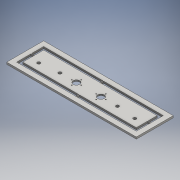
# Autodesk Inventor part: side-UPDATED
Saved by Autodesk Inventor 2,016 (Build 200138000, 138)
## iProperties
Created: 2016-10-15
Part Number: side-UPDATED
Material: Generic
Document SubType Name: Modeling
Designer: Kevin G
Density: 1 g/cm^3
Appearance: Default
Author: Kevin G
Autodesk Inventor part; units mm, degrees
note: some values were not read from the file. Chosen so that the rebuilt part matches the saved one: direction of "Emboss2".
ref_plane "YZ Plane" through (0, 0, 0) normal (1, 0, 0) x (0, 1, 0)
ref_plane "XZ Plane" through (0, 0, 0) normal (0, 1, 0) x (-1, 0, 0)
ref_plane "XY Plane" through (0, 0, 0) normal (0, 0, 1) x (1, 0, 0)
sketch "Sketch1" plane through (0, 0, 0) normal (0, 0, 1) x (1, 0, 0)
  line L0 (-270.2344, -114.33) -> (-270.2344, -13.08)
  circle A0 centre (-227.9995, -79.405) radius 7.5
  circle A1 centre (-134.4524, -69.88) radius 7.5
  circle A2 centre (-54.3408, -69.88) radius 15.875
  circle A3 centre (-54.3408, -46.8612) radius 2.3813
  circle A4 centre (-31.322, -69.88) radius 2.3813
  circle A5 centre (-77.3595, -69.88) radius 2.3813
  circle A6 centre (-54.3408, -92.8987) radius 2.3813
  line L1 (-270.2344, -13.08) -> (5.175, -13.08)
  line L2 (-270.2344, -114.33) -> (5.1968, -114.33)
  line L3 (280.6281, -114.33) -> (280.6281, -13.08)
  line L4 (280.6281, -13.08) -> (5.175, -13.08)
  line L5 (280.6281, -114.33) -> (5.1968, -114.33)
  line L6 (-285.2344, 1.92) -> (295.5844, 1.92)
  line L7 (295.5844, 1.92) -> (295.5844, -129.33)
  line L8 (295.5844, -129.33) -> (-285.2344, -129.33)
  line L9 (-285.2344, -129.33) -> (-285.2344, 1.92)
  line L10 (-59, 1.92) -> (-59, 25.92)
  line L11 (-285.2344, -38) -> (-309.2344, -38)
  line L12 (-43, -129.33) -> (-43, -153.33)
  line L13 (295.5844, -72.2612) -> (319.5844, -72.2612)
  line L14 (-309.2344, 25.92) -> (319.6281, 25.92)
  line L15 (319.6281, 25.92) -> (319.6281, -153.33)
  line L16 (319.6281, -153.33) -> (-309.2344, -153.33)
  line L17 (-309.2344, -153.33) -> (-309.2344, 25.92)
  line L18 (2, -13.08) -> (2, 1.92)
  line L19 (5.175, -13.08) -> (5.175, 1.92)
  line L20 (2, -129.33) -> (2, -114.33)
  line L21 (-285.2344, -56.825) -> (-270.2344, -56.825)
  line L22 (-285.2344, -60) -> (-270.2344, -60)
  line L23 (280.6281, -56.825) -> (295.5844, -56.825)
  line L24 (5.1968, -114.33) -> (5.175, -129.33)
  line L25 (280.6281, -60) -> (295.5844, -60)
  circle A7 centre (238.3931, -79.405) radius 7.5
  circle A8 centre (144.846, -69.88) radius 7.5
  circle A9 centre (64.7344, -69.88) radius 15.875
  circle A10 centre (64.7344, -46.8612) radius 2.3813
  circle A11 centre (41.7157, -69.88) radius 2.3813
  circle A12 centre (87.7532, -69.88) radius 2.3813
  circle A13 centre (64.7344, -92.8987) radius 2.3813
  circle A14 centre (64.7344, -69.88) radius 38.1
  circle A15 centre (-54.3408, -69.88) radius 38.1
  point P0 (0, 0)
  dimension "d4" = 15
  dimension "d7" = 15
  dimension "d9" = 31.75
  dimension "d11" = 4.7625
  dimension "d13" = 4.7625
  dimension "d15" = 23.0188
  dimension "d16" = 4.7625
  dimension "d18" = 4.7625
  dimension "d25" = 550.8625
  dimension "d30" = 24
  dimension "d31" = 24
  dimension "d32" = 24
  dimension "d33" = 24
  dimension "d34" = 3.175
  dimension "d36" = 3.175
  dimension "d50" = 23.0188
  dimension "d51" = 23.0188
  dimension "d52" = 23.0188
  dimension "d53" = 80.1116
  dimension "d54" = 93.5471
  dimension "d56" = 119.0752
  dimension "d57" = 80.1116
  dimension "d60" = 93.5471
  dimension "d61" = 76.2
  dimension "d62" = 76.2
  constraints: 52 end point, 19 point on line, 16 centre point, 6 perpendicular, 5 horizontal, 5 parallel, 3 vertical, 2 coincident, 2 midpoint
  measures "d4" diameter of A0
  measures "d7" diameter of A1
  measures "d9" diameter of A2
  measures "d11" diameter of A3
  measures "d13" diameter of A4
  measures "d15" distance of A2.centre A5.centre
  measures "d16" diameter of A5
  measures "d18" diameter of A6
  measures "d25" distance between parallel lines of L0 L3
  measures "d30" distance of L10.end L10.start
  measures "d31" distance of L11.end L11.start
  measures "d32" distance of L12.start L12.end
  measures "d33" distance of L13.start L13.end
  measures "d34" distance between parallel lines of L19 L18
  measures "d36" distance between parallel lines of L22 L21
  measures "d50" distance of A3.centre A2.centre
  measures "d51" distance of A4.centre A2.centre
  measures "d52" distance of A2.centre A6.centre
  measures "d53" distance of A2.centre A1.centre
  measures "d54" horizontal distance of A0.centre A1.centre
  measures "d56" distance of A9.centre A2.centre
  measures "d57" distance of A8.centre A9.centre
  measures "d60" horizontal distance of A7.centre A8.centre
  measures "d61" diameter of A14
  measures "d62" diameter of A15
extrude "Extrusion2" add sketch "Sketch1" along normal blind 9.525 contours L0 L1 L4 L3 L5 L2 | L22 L9 L21 L0 | L2 L24 L8 L20 | L9 L8 L12 L16 L17 L11 | L8 L7 L6 L10 L14 L15 L16 L12 | L18 L6 L19 L1 | L11 L17 L14 L10 L6 L9 | L3 L23 L7 L25 | A14 | A15
emboss "Emboss2" sketch "Sketch1" operation cut depth 3 direction (0, 0, 1) contours A14 | A15
body "Solid2"
